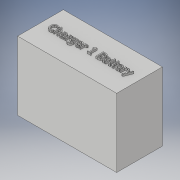
# Autodesk Inventor part: 1 battery charger 2019
Saved by Autodesk Inventor 2019 (Build 230136000, 136)
## iProperties
Created: 2018-12-09
Part Number: 1 battery charger 2019
Material: Generic
Document SubType Name: Modeling
Designer: Tiberus
Density: 1 g/cm^3
Appearance: Default
Author: Tiberus
Autodesk Inventor part; units mm, degrees
ref_plane "YZ Plane" through (0, 0, 0) normal (1, 0, 0) x (0, 1, 0)
ref_plane "XZ Plane" through (0, 0, 0) normal (0, 1, 0) x (-1, 0, 0)
ref_plane "XY Plane" through (0, 0, 0) normal (0, 0, 1) x (1, 0, 0)
sketch "Sketch1" plane through (0, 0, 0) normal (0, 1, 0) x (-1, 0, 0)
  line L0 (0, 0) -> (165.1, 0)
  line L1 (165.1, 0) -> (165.1, -76.2)
  line L2 (165.1, -76.2) -> (0, -76.2)
  line L3 (0, -76.2) -> (0, 0)
  dimension "d0" = 165.1
  dimension "d1" = 76.2
  constraints: 8 end point, 2 parallel, 1 horizontal, 1 perpendicular
  measures "d0" distance of L1.end L2.end
  measures "d1" distance of L0.end L1.end
extrude "Extrusion1" add sketch "Sketch1" along normal blind 114.3
sketch "Sketch3" plane through (0, 114.3, 0) normal (0, 1, 0) x (1, 0, 0)
  line L0 (-164.5039, 75.7893) -> (0, 75.7893) construction
  line L1 (0, 75.7893) -> (0, 0) construction
  line L2 (0, 0) -> (-164.5039, 0) construction
  line L3 (-164.5039, 0) -> (-164.5039, 75.7893) construction
  spline S0 degree 2 poles (-144.3111, 32.8363) (-145.5461, 32.8363) (-147.6353, 33.6699) (-148.3969, 34.5035) knots 0 0 0 1 2 2 2
  spline S1 degree 2 poles (-148.3969, 34.5035) (-149.1585, 35.3269) (-149.9921, 37.7969) (-149.9921, 39.4024) knots 0 0 0 1 2 2 2
  spline S2 degree 2 poles (-149.9921, 39.4024) (-149.9921, 40.9976) (-149.1791, 43.3647) (-148.4072, 44.2395) knots 0 0 0 1 2 2 2
  spline S3 degree 2 poles (-148.4072, 44.2395) (-147.6456, 45.0937) (-145.5667, 45.9891) (-144.2802, 45.9891) knots 0 0 0 1 2 2 2
  spline S4 degree 2 poles (-144.2802, 45.9891) (-143.6421, 45.9891) (-142.5203, 45.8039) (-142.0469, 45.6598) knots 0 0 0 1 2 2 2
  spline S5 degree 2 poles (-142.0469, 45.6598) (-141.6353, 45.526) (-140.781, 45.1452) (-140.3591, 44.9188) knots 0 0 0 1 2 2 2
  line L4 (-140.3591, 44.9188) -> (-140.3591, 42.881)
  line L5 (-140.3591, 42.881) -> (-140.4929, 42.881)
  spline S6 degree 2 poles (-140.4929, 42.881) (-140.7193, 43.0868) (-141.4191, 43.6632) (-141.9234, 43.941) knots 0 0 0 1 2 2 2
  spline S7 degree 2 poles (-141.9234, 43.941) (-142.4071, 44.2086) (-143.5495, 44.5483) (-144.2905, 44.5483) knots 0 0 0 1 2 2 2
  spline S8 degree 2 poles (-144.2905, 44.5483) (-145.1036, 44.5483) (-146.5547, 43.8793) (-147.1002, 43.2412) knots 0 0 0 1 2 2 2
  spline S9 degree 2 poles (-147.1002, 43.2412) (-147.6353, 42.5928) (-148.2323, 40.6271) (-148.2323, 39.4024) knots 0 0 0 1 2 2 2
  spline S10 degree 2 poles (-148.2323, 39.4024) (-148.2323, 38.0953) (-147.6045, 36.212) (-147.059, 35.5636) knots 0 0 0 1 2 2 2
  spline S11 degree 2 poles (-147.059, 35.5636) (-146.5238, 34.9358) (-145.0933, 34.2977) (-144.2905, 34.2977) knots 0 0 0 1 2 2 2
  spline S12 degree 2 poles (-144.2905, 34.2977) (-143.5598, 34.2977) (-142.3145, 34.6579) (-141.8308, 34.9255) knots 0 0 0 1 2 2 2
  spline S13 degree 2 poles (-141.8308, 34.9255) (-141.3677, 35.1931) (-140.6781, 35.7488) (-140.4826, 35.9444) knots 0 0 0 1 2 2 2
  line L6 (-140.4826, 35.9444) -> (-140.3591, 35.9444)
  line L7 (-140.3591, 35.9444) -> (-140.3591, 33.9272)
  spline S14 degree 2 poles (-140.3591, 33.9272) (-140.781, 33.7316) (-141.5221, 33.3714) (-142.0469, 33.2068) knots 0 0 0 1 2 2 2
  spline S15 degree 2 poles (-142.0469, 33.2068) (-142.6027, 33.0215) (-143.5495, 32.8363) (-144.3111, 32.8363) knots 0 0 0 1 2 2 2
  line L8 (-131.4259, 33.0627) -> (-133.0314, 33.0627)
  line L9 (-133.0314, 33.0627) -> (-133.0314, 38.4967)
  spline S16 degree 2 poles (-133.0314, 38.4967) (-133.0314, 39.1554) (-133.1549, 40.2875) (-133.3401, 40.6271) knots 0 0 0 1 2 2 2
  spline S17 degree 2 poles (-133.3401, 40.6271) (-133.5357, 40.9873) (-134.2355, 41.3372) (-134.8324, 41.3372) knots 0 0 0 1 2 2 2
  spline S18 degree 2 poles (-134.8324, 41.3372) (-135.4293, 41.3372) (-136.6952, 40.6992) (-137.3024, 40.1846) knots 0 0 0 1 2 2 2
  line L10 (-137.3024, 40.1846) -> (-137.3024, 33.0627)
  line L11 (-137.3024, 33.0627) -> (-138.908, 33.0627)
  line L12 (-138.908, 33.0627) -> (-138.908, 46.3287)
  line L13 (-138.908, 46.3287) -> (-137.3024, 46.3287)
  line L14 (-137.3024, 46.3287) -> (-137.3024, 41.5328)
  spline S19 degree 2 poles (-137.3024, 41.5328) (-136.582, 42.1812) (-135.1926, 42.8604) (-134.4105, 42.8604) knots 0 0 0 1 2 2 2
  spline S20 degree 2 poles (-134.4105, 42.8604) (-133.0108, 42.8604) (-131.4259, 41.0079) (-131.4259, 39.248) knots 0 0 0 1 2 2 2
  line L15 (-131.4259, 39.248) -> (-131.4259, 33.0627)
  spline S21 degree 2 poles (-123.8614, 34.0713) (-124.057, 33.9272) (-124.7156, 33.4126) (-125.0244, 33.2582) knots 0 0 0 1 2 2 2
  spline S22 degree 2 poles (-125.0244, 33.2582) (-125.4464, 33.0318) (-126.2388, 32.7951) (-126.9592, 32.7951) knots 0 0 0 1 2 2 2
  spline S23 degree 2 poles (-126.9592, 32.7951) (-127.5459, 32.7951) (-128.6059, 33.2376) (-129.0073, 33.639) knots 0 0 0 1 2 2 2
  spline S24 degree 2 poles (-129.0073, 33.639) (-129.3881, 34.0301) (-129.8512, 35.1828) (-129.8512, 35.8209) knots 0 0 0 1 2 2 2
  spline S25 degree 2 poles (-129.8512, 35.8209) (-129.8512, 36.8089) (-129.0176, 38.2086) (-128.1119, 38.6099) knots 0 0 0 1 2 2 2
  spline S26 degree 2 poles (-128.1119, 38.6099) (-127.3092, 38.9804) (-125.1273, 39.2583) (-123.8614, 39.3304) knots 0 0 0 1 2 2 2
  line L16 (-123.8614, 39.3304) -> (-123.8614, 39.6391)
  spline S27 degree 2 poles (-123.8614, 39.6391) (-123.8614, 40.1949) (-124.2011, 40.8844) (-124.5098, 41.0799) knots 0 0 0 1 2 2 2
  spline S28 degree 2 poles (-124.5098, 41.0799) (-124.8186, 41.2755) (-125.7037, 41.399) (-126.1771, 41.399) knots 0 0 0 1 2 2 2
  spline S29 degree 2 poles (-126.1771, 41.399) (-126.7328, 41.399) (-128.2354, 41.0697) (-128.9867, 40.7506) knots 0 0 0 1 2 2 2
  line L17 (-128.9867, 40.7506) -> (-129.0793, 40.7506)
  line L18 (-129.0793, 40.7506) -> (-129.0793, 42.387)
  spline S30 degree 2 poles (-129.0793, 42.387) (-128.6368, 42.5105) (-126.9798, 42.8192) (-126.1668, 42.8192) knots 0 0 0 1 2 2 2
  spline S31 degree 2 poles (-126.1668, 42.8192) (-125.1788, 42.8192) (-123.8306, 42.5105) (-123.2954, 42.1091) knots 0 0 0 1 2 2 2
  spline S32 degree 2 poles (-123.2954, 42.1091) (-122.7705, 41.718) (-122.2559, 40.4727) (-122.2559, 39.5774) knots 0 0 0 1 2 2 2
  line L19 (-122.2559, 39.5774) -> (-122.2559, 33.0627)
  line L20 (-122.2559, 33.0627) -> (-123.8614, 33.0627)
  line L21 (-123.8614, 33.0627) -> (-123.8614, 34.0713)
  line L22 (-123.8614, 35.4092) -> (-123.8614, 38.0542)
  spline S33 degree 2 poles (-123.8614, 38.0542) (-124.4378, 38.0027) (-126.1771, 37.8278) (-126.7225, 37.6631) knots 0 0 0 1 2 2 2
  spline S34 degree 2 poles (-126.7225, 37.6631) (-127.3606, 37.4675) (-128.1943, 36.6545) (-128.1943, 35.9341) knots 0 0 0 1 2 2 2
  spline S35 degree 2 poles (-128.1943, 35.9341) (-128.1943, 35.1107) (-127.268, 34.2771) (-126.3829, 34.2771) knots 0 0 0 1 2 2 2
  spline S36 degree 2 poles (-126.3829, 34.2771) (-125.6316, 34.2771) (-124.3966, 34.9255) (-123.8614, 35.4092) knots 0 0 0 1 2 2 2
  line L23 (-114.9488, 40.8741) -> (-115.0311, 40.8741)
  spline S37 degree 2 poles (-115.0311, 40.8741) (-115.2164, 40.9256) (-115.6178, 40.9462) (-115.8956, 40.9462) knots 0 0 0 1 2 2 2
  spline S38 degree 2 poles (-115.8956, 40.9462) (-116.544, 40.9462) (-117.8202, 40.3801) (-118.3965, 39.8244) knots 0 0 0 1 2 2 2
  line L24 (-118.3965, 39.8244) -> (-118.3965, 33.0627)
  line L25 (-118.3965, 33.0627) -> (-120.002, 33.0627)
  line L26 (-120.002, 33.0627) -> (-120.002, 42.5928)
  line L27 (-120.002, 42.5928) -> (-118.3965, 42.5928)
  line L28 (-118.3965, 42.5928) -> (-118.3965, 41.1726)
  spline S39 degree 2 poles (-118.3965, 41.1726) (-117.5217, 41.9547) (-116.2147, 42.5928) (-115.5972, 42.5928) knots 0 0 0 1 2 2 2
  spline S40 degree 2 poles (-115.5972, 42.5928) (-115.3502, 42.5928) (-115.1032, 42.5722) (-114.9488, 42.5414) knots 0 0 0 1 2 2 2
  line L29 (-114.9488, 42.5414) -> (-114.9488, 40.8741)
  spline S41 degree 2 poles (-113.3639, 31.5395) (-113.1992, 31.4675) (-112.5714, 31.241) (-112.17, 31.1484) knots 0 0 0 1 2 2 2
  spline S42 degree 2 poles (-112.17, 31.1484) (-111.7275, 31.0352) (-110.9762, 30.9014) (-110.5336, 30.9014) knots 0 0 0 1 2 2 2
  spline S43 degree 2 poles (-110.5336, 30.9014) (-109.7926, 30.9014) (-108.7635, 31.2925) (-108.4753, 31.6424) knots 0 0 0 1 2 2 2
  spline S44 degree 2 poles (-108.4753, 31.6424) (-108.1974, 31.9923) (-107.9813, 32.9083) (-107.9813, 33.4949) knots 0 0 0 1 2 2 2
  line L30 (-107.9813, 33.4949) -> (-107.9813, 34.3286)
  spline S45 degree 2 poles (-107.9813, 34.3286) (-108.6297, 33.7625) (-109.875, 33.2274) (-110.8115, 33.2274) knots 0 0 0 1 2 2 2
  spline S46 degree 2 poles (-110.8115, 33.2274) (-112.4376, 33.2274) (-114.3622, 35.6459) (-114.3622, 37.9204) knots 0 0 0 1 2 2 2
  spline S47 degree 2 poles (-114.3622, 37.9204) (-114.3622, 39.1039) (-113.6932, 40.9359) (-113.1374, 41.5842) knots 0 0 0 1 2 2 2
  spline S48 degree 2 poles (-113.1374, 41.5842) (-112.6023, 42.1915) (-111.1306, 42.8604) (-110.3484, 42.8604) knots 0 0 0 1 2 2 2
  spline S49 degree 2 poles (-110.3484, 42.8604) (-109.6074, 42.8604) (-108.5268, 42.5105) (-107.9813, 42.1915) knots 0 0 0 1 2 2 2
  line L31 (-107.9813, 42.1915) -> (-107.8887, 42.5928)
  line L32 (-107.8887, 42.5928) -> (-106.3758, 42.5928)
  line L33 (-106.3758, 42.5928) -> (-106.3758, 34.1536)
  spline S50 degree 2 poles (-106.3758, 34.1536) (-106.3758, 31.7248) (-108.4856, 29.4606) (-110.6571, 29.4606) knots 0 0 0 1 2 2 2
  spline S51 degree 2 poles (-110.6571, 29.4606) (-111.357, 29.4606) (-112.8184, 29.687) (-113.4462, 29.8722) knots 0 0 0 1 2 2 2
  line L34 (-113.4462, 29.8722) -> (-113.4462, 31.5395)
  line L35 (-113.4462, 31.5395) -> (-113.3639, 31.5395)
  line L36 (-107.9813, 35.6459) -> (-107.9813, 40.8844)
  spline S52 degree 2 poles (-107.9813, 40.8844) (-108.5782, 41.1726) (-109.5868, 41.4196) (-110.0911, 41.4196) knots 0 0 0 1 2 2 2
  spline S53 degree 2 poles (-110.0911, 41.4196) (-111.3055, 41.4196) (-112.7052, 39.6288) (-112.7052, 37.9513) knots 0 0 0 1 2 2 2
  spline S54 degree 2 poles (-112.7052, 37.9513) (-112.7052, 36.3663) (-111.6451, 34.7094) (-110.4513, 34.7094) knots 0 0 0 1 2 2 2
  spline S55 degree 2 poles (-110.4513, 34.7094) (-109.8235, 34.7094) (-108.5062, 35.2034) (-107.9813, 35.6459) knots 0 0 0 1 2 2 2
  spline S56 degree 2 poles (-99.9126, 32.8466) (-102.1973, 32.8466) (-104.7085, 35.4092) (-104.7085, 37.7763) knots 0 0 0 1 2 2 2
  spline S57 degree 2 poles (-104.7085, 37.7763) (-104.7085, 40.1022) (-102.2694, 42.8604) (-100.3037, 42.8604) knots 0 0 0 1 2 2 2
  spline S58 degree 2 poles (-100.3037, 42.8604) (-99.4186, 42.8604) (-98.0498, 42.3458) (-97.5455, 41.8004) knots 0 0 0 1 2 2 2
  spline S59 degree 2 poles (-97.5455, 41.8004) (-97.0309, 41.2549) (-96.4854, 39.6803) (-96.4854, 38.5379) knots 0 0 0 1 2 2 2
  line L37 (-96.4854, 38.5379) -> (-96.4854, 37.6631)
  line L38 (-96.4854, 37.6631) -> (-103.0824, 37.6631)
  spline S60 degree 2 poles (-103.0824, 37.6631) (-103.0824, 36.0061) (-101.4152, 34.2462) (-99.9332, 34.2462) knots 0 0 0 1 2 2 2
  spline S61 degree 2 poles (-99.9332, 34.2462) (-99.4083, 34.2462) (-98.3894, 34.4829) (-97.9777, 34.6682) knots 0 0 0 1 2 2 2
  spline S62 degree 2 poles (-97.9777, 34.6682) (-97.5455, 34.874) (-96.9486, 35.2342) (-96.753, 35.3989) knots 0 0 0 1 2 2 2
  line L39 (-96.753, 35.3989) -> (-96.6604, 35.3989)
  line L40 (-96.6604, 35.3989) -> (-96.6604, 33.6493)
  spline S63 degree 2 poles (-96.6604, 33.6493) (-96.9383, 33.5361) (-97.7822, 33.2068) (-98.1115, 33.1141) knots 0 0 0 1 2 2 2
  spline S64 degree 2 poles (-98.1115, 33.1141) (-98.5746, 32.9804) (-99.3362, 32.8466) (-99.9126, 32.8466) knots 0 0 0 1 2 2 2
  spline S65 degree 2 poles (-98.0498, 38.8878) (-98.0703, 39.5362) (-98.3379, 40.483) (-98.5952, 40.8021) knots 0 0 0 1 2 2 2
  spline S66 degree 2 poles (-98.5952, 40.8021) (-98.8731, 41.1623) (-99.7479, 41.5431) (-100.3963, 41.5431) knots 0 0 0 1 2 2 2
  spline S67 degree 2 poles (-100.3963, 41.5431) (-101.0344, 41.5431) (-101.9297, 41.1623) (-102.3003, 40.7918) knots 0 0 0 1 2 2 2
  spline S68 degree 2 poles (-102.3003, 40.7918) (-102.6605, 40.411) (-103.031, 39.495) (-103.0824, 38.8878) knots 0 0 0 1 2 2 2
  line L41 (-103.0824, 38.8878) -> (-98.0498, 38.8878)
  line L42 (-89.8061, 40.8741) -> (-89.8884, 40.8741)
  spline S69 degree 2 poles (-89.8884, 40.8741) (-90.0737, 40.9256) (-90.475, 40.9462) (-90.7529, 40.9462) knots 0 0 0 1 2 2 2
  spline S70 degree 2 poles (-90.7529, 40.9462) (-91.4013, 40.9462) (-92.6775, 40.3801) (-93.2538, 39.8244) knots 0 0 0 1 2 2 2
  line L43 (-93.2538, 39.8244) -> (-93.2538, 33.0627)
  line L44 (-93.2538, 33.0627) -> (-94.8593, 33.0627)
  line L45 (-94.8593, 33.0627) -> (-94.8593, 42.5928)
  line L46 (-94.8593, 42.5928) -> (-93.2538, 42.5928)
  line L47 (-93.2538, 42.5928) -> (-93.2538, 41.1726)
  spline S71 degree 2 poles (-93.2538, 41.1726) (-92.379, 41.9547) (-91.072, 42.5928) (-90.4545, 42.5928) knots 0 0 0 1 2 2 2
  spline S72 degree 2 poles (-90.4545, 42.5928) (-90.2075, 42.5928) (-89.9605, 42.5722) (-89.8061, 42.5414) knots 0 0 0 1 2 2 2
  line L48 (-89.8061, 42.5414) -> (-89.8061, 40.8741)
  line L49 (-76.149, 33.0627) -> (-82.3446, 33.0627)
  line L50 (-82.3446, 33.0627) -> (-82.3446, 34.3594)
  line L51 (-82.3446, 34.3594) -> (-80.0392, 34.3594)
  line L52 (-80.0392, 34.3594) -> (-80.0392, 42.8707)
  line L53 (-80.0392, 42.8707) -> (-82.3446, 42.8707)
  line L54 (-82.3446, 42.8707) -> (-82.3446, 44.0337)
  spline S73 degree 2 poles (-82.3446, 44.0337) (-81.0375, 44.0337) (-79.8025, 44.7747) (-79.7202, 45.8039) knots 0 0 0 1 2 2 2
  line L55 (-79.7202, 45.8039) -> (-78.4028, 45.8039)
  line L56 (-78.4028, 45.8039) -> (-78.4028, 34.3594)
  line L57 (-78.4028, 34.3594) -> (-76.149, 34.3594)
  line L58 (-76.149, 34.3594) -> (-76.149, 33.0627)
  spline S74 degree 2 poles (-59.3837, 36.9633) (-59.3837, 36.0164) (-60.1041, 34.5653) (-60.7011, 34.0919) knots 0 0 0 1 2 2 2
  spline S75 degree 2 poles (-60.7011, 34.0919) (-61.4215, 33.5361) (-63.0579, 33.0627) (-64.3546, 33.0627) knots 0 0 0 1 2 2 2
  line L59 (-64.3546, 33.0627) -> (-67.9979, 33.0627)
  line L60 (-67.9979, 33.0627) -> (-67.9979, 45.7627)
  line L61 (-67.9979, 45.7627) -> (-64.6325, 45.7627)
  spline S76 degree 2 poles (-64.6325, 45.7627) (-63.274, 45.7627) (-61.9155, 45.5877) (-61.298, 45.2481) knots 0 0 0 1 2 2 2
  spline S77 degree 2 poles (-61.298, 45.2481) (-60.6084, 44.8879) (-59.9806, 43.7043) (-59.9806, 42.9016) knots 0 0 0 1 2 2 2
  spline S78 degree 2 poles (-59.9806, 42.9016) (-59.9806, 42.0062) (-60.9275, 40.5859) (-61.7611, 40.1846) knots 0 0 0 1 2 2 2
  line L62 (-61.7611, 40.1846) -> (-61.7611, 40.1228)
  spline S79 degree 2 poles (-61.7611, 40.1228) (-60.629, 39.8141) (-59.3837, 38.1777) (-59.3837, 36.9633) knots 0 0 0 1 2 2 2
  spline S80 degree 2 poles (-61.1436, 36.8912) (-61.1436, 37.6116) (-61.5553, 38.5379) (-62.1728, 38.8672) knots 0 0 0 1 2 2 2
  spline S81 degree 2 poles (-62.1728, 38.8672) (-62.5742, 39.0731) (-63.521, 39.1966) (-64.3958, 39.1966) knots 0 0 0 1 2 2 2
  line L63 (-64.3958, 39.1966) -> (-66.3101, 39.1966)
  line L64 (-66.3101, 39.1966) -> (-66.3101, 34.5035)
  line L65 (-66.3101, 34.5035) -> (-64.9413, 34.5035)
  spline S82 degree 2 poles (-64.9413, 34.5035) (-63.8298, 34.5035) (-62.5536, 34.7094) (-62.0596, 35.0387) knots 0 0 0 1 2 2 2
  spline S83 degree 2 poles (-62.0596, 35.0387) (-61.5862, 35.3783) (-61.1436, 36.2222) (-61.1436, 36.8912) knots 0 0 0 1 2 2 2
  spline S84 degree 2 poles (-61.7405, 42.6649) (-61.7405, 43.1177) (-62.0493, 43.797) (-62.3889, 43.9925) knots 0 0 0 1 2 2 2
  spline S85 degree 2 poles (-62.3889, 43.9925) (-62.8006, 44.2189) (-63.7989, 44.3218) (-64.6943, 44.3218) knots 0 0 0 1 2 2 2
  line L66 (-64.6943, 44.3218) -> (-66.3101, 44.3218)
  line L67 (-66.3101, 44.3218) -> (-66.3101, 40.6065)
  line L68 (-66.3101, 40.6065) -> (-64.3958, 40.6065)
  spline S86 degree 2 poles (-64.3958, 40.6065) (-63.6033, 40.6065) (-62.852, 40.7712) (-62.4507, 41.0285) knots 0 0 0 1 2 2 2
  spline S87 degree 2 poles (-62.4507, 41.0285) (-62.0596, 41.2755) (-61.7405, 42.068) (-61.7405, 42.6649) knots 0 0 0 1 2 2 2
  spline S88 degree 2 poles (-52.5191, 34.0713) (-52.7147, 33.9272) (-53.3733, 33.4126) (-53.6821, 33.2582) knots 0 0 0 1 2 2 2
  spline S89 degree 2 poles (-53.6821, 33.2582) (-54.1041, 33.0318) (-54.8965, 32.7951) (-55.6169, 32.7951) knots 0 0 0 1 2 2 2
  spline S90 degree 2 poles (-55.6169, 32.7951) (-56.2036, 32.7951) (-57.2636, 33.2376) (-57.665, 33.639) knots 0 0 0 1 2 2 2
  spline S91 degree 2 poles (-57.665, 33.639) (-58.0458, 34.0301) (-58.5089, 35.1828) (-58.5089, 35.8209) knots 0 0 0 1 2 2 2
  spline S92 degree 2 poles (-58.5089, 35.8209) (-58.5089, 36.8089) (-57.6753, 38.2086) (-56.7696, 38.6099) knots 0 0 0 1 2 2 2
  spline S93 degree 2 poles (-56.7696, 38.6099) (-55.9669, 38.9804) (-53.785, 39.2583) (-52.5191, 39.3304) knots 0 0 0 1 2 2 2
  line L69 (-52.5191, 39.3304) -> (-52.5191, 39.6391)
  spline S94 degree 2 poles (-52.5191, 39.6391) (-52.5191, 40.1949) (-52.8588, 40.8844) (-53.1675, 41.0799) knots 0 0 0 1 2 2 2
  spline S95 degree 2 poles (-53.1675, 41.0799) (-53.4763, 41.2755) (-54.3614, 41.399) (-54.8348, 41.399) knots 0 0 0 1 2 2 2
  spline S96 degree 2 poles (-54.8348, 41.399) (-55.3905, 41.399) (-56.8931, 41.0697) (-57.6444, 40.7506) knots 0 0 0 1 2 2 2
  line L70 (-57.6444, 40.7506) -> (-57.737, 40.7506)
  line L71 (-57.737, 40.7506) -> (-57.737, 42.387)
  spline S97 degree 2 poles (-57.737, 42.387) (-57.2945, 42.5105) (-55.6375, 42.8192) (-54.8245, 42.8192) knots 0 0 0 1 2 2 2
  spline S98 degree 2 poles (-54.8245, 42.8192) (-53.8365, 42.8192) (-52.4883, 42.5105) (-51.9531, 42.1091) knots 0 0 0 1 2 2 2
  spline S99 degree 2 poles (-51.9531, 42.1091) (-51.4282, 41.718) (-50.9136, 40.4727) (-50.9136, 39.5774) knots 0 0 0 1 2 2 2
  line L72 (-50.9136, 39.5774) -> (-50.9136, 33.0627)
  line L73 (-50.9136, 33.0627) -> (-52.5191, 33.0627)
  line L74 (-52.5191, 33.0627) -> (-52.5191, 34.0713)
  line L75 (-52.5191, 35.4092) -> (-52.5191, 38.0542)
  spline S100 degree 2 poles (-52.5191, 38.0542) (-53.0955, 38.0027) (-54.8348, 37.8278) (-55.3802, 37.6631) knots 0 0 0 1 2 2 2
  spline S101 degree 2 poles (-55.3802, 37.6631) (-56.0183, 37.4675) (-56.852, 36.6545) (-56.852, 35.9341) knots 0 0 0 1 2 2 2
  spline S102 degree 2 poles (-56.852, 35.9341) (-56.852, 35.1107) (-55.9257, 34.2771) (-55.0406, 34.2771) knots 0 0 0 1 2 2 2
  spline S103 degree 2 poles (-55.0406, 34.2771) (-54.2893, 34.2771) (-53.0543, 34.9255) (-52.5191, 35.4092) knots 0 0 0 1 2 2 2
  spline S104 degree 2 poles (-45.778, 32.8774) (-47.0851, 32.8774) (-48.5568, 34.3697) (-48.5568, 35.9855) knots 0 0 0 1 2 2 2
  line L76 (-48.5568, 35.9855) -> (-48.5568, 41.2652)
  line L77 (-48.5568, 41.2652) -> (-49.6374, 41.2652)
  line L78 (-49.6374, 41.2652) -> (-49.6374, 42.5928)
  line L79 (-49.6374, 42.5928) -> (-48.5568, 42.5928)
  line L80 (-48.5568, 42.5928) -> (-48.5568, 45.3304)
  line L81 (-48.5568, 45.3304) -> (-46.9513, 45.3304)
  line L82 (-46.9513, 45.3304) -> (-46.9513, 42.5928)
  line L83 (-46.9513, 42.5928) -> (-43.9976, 42.5928)
  line L84 (-43.9976, 42.5928) -> (-43.9976, 41.2652)
  line L85 (-43.9976, 41.2652) -> (-46.9513, 41.2652)
  line L86 (-46.9513, 41.2652) -> (-46.9513, 36.7265)
  spline S105 degree 2 poles (-46.9513, 36.7265) (-46.9513, 36.0061) (-46.8998, 35.2137) (-46.7249, 34.874) knots 0 0 0 1 2 2 2
  spline S106 degree 2 poles (-46.7249, 34.874) (-46.5808, 34.5756) (-45.9324, 34.2771) (-45.3767, 34.2771) knots 0 0 0 1 2 2 2
  spline S107 degree 2 poles (-45.3767, 34.2771) (-44.9856, 34.2771) (-44.2549, 34.5138) (-44.0902, 34.5859) knots 0 0 0 1 2 2 2
  line L87 (-44.0902, 34.5859) -> (-43.9976, 34.5859)
  line L88 (-43.9976, 34.5859) -> (-43.9976, 33.145)
  spline S108 degree 2 poles (-43.9976, 33.145) (-44.4504, 33.0215) (-45.3767, 32.8774) (-45.778, 32.8774) knots 0 0 0 1 2 2 2
  spline S109 degree 2 poles (-39.9323, 32.8774) (-41.2394, 32.8774) (-42.7111, 34.3697) (-42.7111, 35.9855) knots 0 0 0 1 2 2 2
  line L89 (-42.7111, 35.9855) -> (-42.7111, 41.2652)
  line L90 (-42.7111, 41.2652) -> (-43.7917, 41.2652)
  line L91 (-43.7917, 41.2652) -> (-43.7917, 42.5928)
  line L92 (-43.7917, 42.5928) -> (-42.7111, 42.5928)
  line L93 (-42.7111, 42.5928) -> (-42.7111, 45.3304)
  line L94 (-42.7111, 45.3304) -> (-41.1056, 45.3304)
  line L95 (-41.1056, 45.3304) -> (-41.1056, 42.5928)
  line L96 (-41.1056, 42.5928) -> (-38.1519, 42.5928)
  line L97 (-38.1519, 42.5928) -> (-38.1519, 41.2652)
  line L98 (-38.1519, 41.2652) -> (-41.1056, 41.2652)
  line L99 (-41.1056, 41.2652) -> (-41.1056, 36.7265)
  spline S110 degree 2 poles (-41.1056, 36.7265) (-41.1056, 36.0061) (-41.0541, 35.2137) (-40.8792, 34.874) knots 0 0 0 1 2 2 2
  spline S111 degree 2 poles (-40.8792, 34.874) (-40.7351, 34.5756) (-40.0867, 34.2771) (-39.531, 34.2771) knots 0 0 0 1 2 2 2
  spline S112 degree 2 poles (-39.531, 34.2771) (-39.1399, 34.2771) (-38.4092, 34.5138) (-38.2445, 34.5859) knots 0 0 0 1 2 2 2
  line L100 (-38.2445, 34.5859) -> (-38.1519, 34.5859)
  line L101 (-38.1519, 34.5859) -> (-38.1519, 33.145)
  spline S113 degree 2 poles (-38.1519, 33.145) (-38.6047, 33.0215) (-39.531, 32.8774) (-39.9323, 32.8774) knots 0 0 0 1 2 2 2
  spline S114 degree 2 poles (-32.831, 32.8466) (-35.1158, 32.8466) (-37.627, 35.4092) (-37.627, 37.7763) knots 0 0 0 1 2 2 2
  spline S115 degree 2 poles (-37.627, 37.7763) (-37.627, 40.1022) (-35.1879, 42.8604) (-33.2221, 42.8604) knots 0 0 0 1 2 2 2
  spline S116 degree 2 poles (-33.2221, 42.8604) (-32.337, 42.8604) (-30.9682, 42.3458) (-30.4639, 41.8004) knots 0 0 0 1 2 2 2
  spline S117 degree 2 poles (-30.4639, 41.8004) (-29.9494, 41.2549) (-29.4039, 39.6803) (-29.4039, 38.5379) knots 0 0 0 1 2 2 2
  line L102 (-29.4039, 38.5379) -> (-29.4039, 37.6631)
  line L103 (-29.4039, 37.6631) -> (-36.0009, 37.6631)
  spline S118 degree 2 poles (-36.0009, 37.6631) (-36.0009, 36.0061) (-34.3336, 34.2462) (-32.8516, 34.2462) knots 0 0 0 1 2 2 2
  spline S119 degree 2 poles (-32.8516, 34.2462) (-32.3268, 34.2462) (-31.3079, 34.4829) (-30.8962, 34.6682) knots 0 0 0 1 2 2 2
  spline S120 degree 2 poles (-30.8962, 34.6682) (-30.4639, 34.874) (-29.867, 35.2342) (-29.6715, 35.3989) knots 0 0 0 1 2 2 2
  line L104 (-29.6715, 35.3989) -> (-29.5789, 35.3989)
  line L105 (-29.5789, 35.3989) -> (-29.5789, 33.6493)
  spline S121 degree 2 poles (-29.5789, 33.6493) (-29.8567, 33.5361) (-30.7007, 33.2068) (-31.03, 33.1141) knots 0 0 0 1 2 2 2
  spline S122 degree 2 poles (-31.03, 33.1141) (-31.4931, 32.9804) (-32.2547, 32.8466) (-32.831, 32.8466) knots 0 0 0 1 2 2 2
  spline S123 degree 2 poles (-30.9682, 38.8878) (-30.9888, 39.5362) (-31.2564, 40.483) (-31.5137, 40.8021) knots 0 0 0 1 2 2 2
  spline S124 degree 2 poles (-31.5137, 40.8021) (-31.7916, 41.1623) (-32.6664, 41.5431) (-33.3148, 41.5431) knots 0 0 0 1 2 2 2
  spline S125 degree 2 poles (-33.3148, 41.5431) (-33.9528, 41.5431) (-34.8482, 41.1623) (-35.2187, 40.7918) knots 0 0 0 1 2 2 2
  spline S126 degree 2 poles (-35.2187, 40.7918) (-35.5789, 40.411) (-35.9494, 39.495) (-36.0009, 38.8878) knots 0 0 0 1 2 2 2
  line L106 (-36.0009, 38.8878) -> (-30.9682, 38.8878)
  line L107 (-22.7246, 40.8741) -> (-22.8069, 40.8741)
  spline S127 degree 2 poles (-22.8069, 40.8741) (-22.9921, 40.9256) (-23.3935, 40.9462) (-23.6714, 40.9462) knots 0 0 0 1 2 2 2
  spline S128 degree 2 poles (-23.6714, 40.9462) (-24.3198, 40.9462) (-25.596, 40.3801) (-26.1723, 39.8244) knots 0 0 0 1 2 2 2
  line L108 (-26.1723, 39.8244) -> (-26.1723, 33.0627)
  line L109 (-26.1723, 33.0627) -> (-27.7778, 33.0627)
  line L110 (-27.7778, 33.0627) -> (-27.7778, 42.5928)
  line L111 (-27.7778, 42.5928) -> (-26.1723, 42.5928)
  line L112 (-26.1723, 42.5928) -> (-26.1723, 41.1726)
  spline S129 degree 2 poles (-26.1723, 41.1726) (-25.2975, 41.9547) (-23.9904, 42.5928) (-23.3729, 42.5928) knots 0 0 0 1 2 2 2
  spline S130 degree 2 poles (-23.3729, 42.5928) (-23.1259, 42.5928) (-22.8789, 42.5722) (-22.7246, 42.5414) knots 0 0 0 1 2 2 2
  line L113 (-22.7246, 42.5414) -> (-22.7246, 40.8741)
  line L114 (-13.9972, 42.5928) -> (-19.1225, 29.5532)
  line L115 (-19.1225, 29.5532) -> (-20.8412, 29.5532)
  line L116 (-20.8412, 29.5532) -> (-19.1327, 33.5258)
  line L117 (-19.1327, 33.5258) -> (-22.5908, 42.5928)
  line L118 (-22.5908, 42.5928) -> (-20.8618, 42.5928)
  line L119 (-20.8618, 42.5928) -> (-18.258, 35.5327)
  line L120 (-18.258, 35.5327) -> (-15.6644, 42.5928)
  line L121 (-15.6644, 42.5928) -> (-13.9972, 42.5928)
  constraints: 1 coincident, 2 other
emboss "Emboss1" sketch "Sketch3" operation add depth 3.175 direction (0, -1, 0)
body "Solid1"
